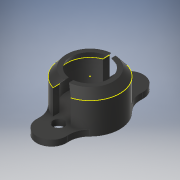
# Autodesk Inventor part: CasterEnclosure
Saved by Autodesk Inventor 2018 (Build 220112000, 112)
## iProperties
Created: 2018-01-18
Part Number: CasterEnclosure
Material: ABS Plastic
Document SubType Name: Modeling
Designer: mmarkle
Density: 1.06 g/cm^3
Appearance: Smooth - Black
Author: mmarkle
Autodesk Inventor part; units mm, degrees
ref_plane "YZ Plane" through (0, 0, 0) normal (1, 0, 0) x (0, 1, 0)
ref_plane "XZ Plane" through (0, 0, 0) normal (0, 1, 0) x (-1, 0, 0)
sketch "Sketch1" plane through (0, 0, 0) normal (0, 1, 0) x (-1, 0, 0)
  arc A0 (-4.4691, 4.5111) -> (4.4691, 4.5111) centre (0, 0) ccw
  arc A1 (3.1656, 8.0108) -> (-3.1656, 8.0108) centre (0, 8.255) ccw
  circle A2 centre (0, -8.255) radius 3.175
  line L0 (0, 0) -> (3.175, 0)
  arc A3 (3.1656, 8.0108) -> (4.4691, 4.5111) centre (7.5974, 7.6688) ccw
  arc A4 (-4.4691, 4.5111) -> (-3.1656, 8.0108) centre (-7.5974, 7.6688) ccw
  arc A5 (-3.1656, -8.0108) -> (-4.4691, -4.5111) centre (-7.5974, -7.6688) ccw
  arc A6 (4.4691, -4.5111) -> (3.1656, -8.0108) centre (7.5974, -7.6688) ccw
  dimension "d0" = 12.7
  dimension "d2" = 6.35
  dimension "d4" = 6.35
  dimension "d5" = 8.89
  dimension "d6" = 16.51
  constraints: 16 point on circle, 8 tangent, 7 centre point, 3 equal radius, 2 end point, 1 coincident, 1 horizontal, 1 symmetric about line, 1 vertical alignment
  measures "d0" diameter of A0
  measures "d2" diameter of A1
  measures "d4" diameter of A2
  measures "d5" diameter of A3
  measures "d6" distance of A1.centre A2.centre
extrude "Extrusion1" add sketch "Sketch1" along normal blind 1.27
sketch "Sketch2" plane through (0, 1.27, 0) normal (0, 1, 0) x (1, 0, 0)
  line L0 (1.905, -7.3814) -> (-1.905, -7.3814)
  line L1 (-1.905, -7.3814) -> (-1.905, 7.3814)
  line L2 (-1.905, 7.3814) -> (1.905, 7.3814)
  line L3 (1.905, 7.3814) -> (1.905, -7.3814)
  line L4 (1.905, -7.3814) -> (-1.905, 7.3814) construction
  line L5 (-1.905, -7.3814) -> (1.905, 7.3814) construction
  arc A0 (1.905, -4.6407) -> (1.905, 4.6407) centre (0, 0) ccw
  arc A1 (-1.905, 4.6407) -> (-1.905, -4.6407) centre (0, 0) ccw
  arc A2 (1.905, -6.0575) -> (1.905, 6.0575) centre (0, 0) ccw
  arc A3 (-1.905, 6.0575) -> (-1.905, -6.0575) centre (0, 0) ccw
  dimension "d11" = 3.81
  dimension "d34" = 5.0165
  dimension "d35" = 6.35
  dimension "d36" = 5.0165
  dimension "d37" = 6.35
  constraints: 12 end point, 8 point on circle, 8 point on line, 4 centre point, 2 coincident, 2 midpoint, 2 parallel, 1 horizontal, 1 perpendicular
  measures "d11" distance of L1.end L2.end
  measures "d34" radius of A1
  measures "d35" radius of A3
  measures "d36" radius of A0
  measures "d37" radius of A2
extrude "Extrusion2" add sketch "Sketch2" along normal blind 5.3975 contours L3 A0 A2 | A3 L1 A1
sketch "Sketch3" plane through (0, 6.6675, 0) normal (0, 1, 0) x (1, 0, 0)
  arc A0 (-1.905, 4.6407) -> (-1.905, -4.6407) centre (0, 0) ccw projected
  line L0 (-1.905, 4.6407) -> (-1.905, 6.0575) projected
  arc A1 (-1.905, 6.0575) -> (-1.905, -6.0575) centre (0, 0) ccw projected
  line L1 (-1.905, -6.0575) -> (-1.905, -4.6407) projected
  line L2 (1.905, -4.6407) -> (1.905, -6.0575) projected
  arc A2 (1.905, -6.0575) -> (1.905, 6.0575) centre (0, 0) ccw projected
  line L3 (1.905, 6.0575) -> (1.905, 4.6407) projected
  arc A3 (1.905, -4.6407) -> (1.905, 4.6407) centre (0, 0) ccw projected
ref_plane "Work Plane1" through (0, 8.255, 0) normal (0, 1, 0) x (1, 0, 0)
sketch "Sketch4" plane through (0, 8.255, 0) normal (0, 1, 0) x (1, 0, 0)
  arc A0 (0.508, -4.9907) -> (0.508, 4.9907) centre (0, 0) ccw
  arc A1 (0.508, -4.0961) -> (0.508, 4.0961) centre (0, 0) ccw
  line L0 (0.508, -4.9907) -> (0.508, -4.0961)
  line L1 (0.508, 4.0961) -> (0.508, 4.9907)
  constraints: 4 end point, 4 point on circle, 2 centre point, 2 coincident
sketch "Sketch5" plane through (0, 8.255, 0) normal (0, 1, 0) x (1, 0, 0)
  line L0 (-0.508, -4.0961) -> (-0.508, -4.9907) projected
  arc A0 (-0.508, 4.0961) -> (-0.508, -4.0961) centre (0, 0) ccw projected
  arc A1 (-0.508, 4.9907) -> (-0.508, -4.9907) centre (0, 0) ccw projected
  line L1 (-0.508, 4.0961) -> (-0.508, 4.9907)
  constraints: 2 end point, 1 vertical
loft "Loft1" add profiles "Sketch4" section 1 edges at (1.905, 6.6675, 5.3491) (6.35, 6.6675, 0) (1.905, 6.6675, -5.3491) (5.0165, 6.6675, 0)
loft "Loft2" add profiles "Sketch5" section 1 edges at (-5.0165, 6.6675, 0) (-1.905, 6.6675, -5.3491) (-6.35, 6.6675, 0) (-1.905, 6.6675, 5.3491)
sketch "Sketch6" plane through (0, 1.27, 0) normal (0, 1, 0) x (1, 0, 0)
  line L0 (0, 0) -> (-3.0006, 0)
  point P0 (0, -6.731)
  point P1 (0, 6.731)
  dimension "d26" = 13.462
  constraints: 2 end point, 2 vertical alignment, 1 horizontal, 1 symmetric about line
  measures "d26" distance of point (0, 6.731) point (0, -6.731)
hole "Hole1" at (0, 1.27, 6.731) at (0, 1.27, -6.731) direction (0, -1, 0) diameter 2.4384 end through all clearance for "Flat Head Machine Screw (82)" size "#2" standard "Ansi Unified Screw Threads"
body "Solid1"
